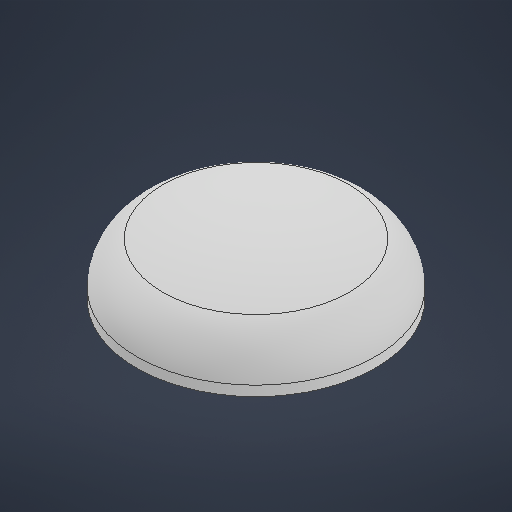
# Autodesk Inventor part: Fuel Cap Outlet
Saved by Autodesk Inventor 2026 (Build 300175050, 175E)
## iProperties
Created: 2026-03-18
Part Number: Fuel Cap Outlet
Material: Generic
Document SubType Name: Modeling
Designer: jackr
Density: 1 g/cm^3
Appearance: Default
Author: jackr
Autodesk Inventor part; units mm, degrees
ref_plane "YZ Plane" through (0, 0, 0) normal (1, 0, 0) x (0, 1, 0)
ref_plane "XZ Plane" through (0, 0, 0) normal (0, 1, 0) x (-1, 0, 0)
ref_plane "XY Plane" through (0, 0, 0) normal (0, 0, 1) x (1, 0, 0)
sketch "Sketch1" plane through (0, 0, 0) normal (0, 0, 1) x (1, 0, 0)
  arc A0 (0, 81.5967) -> (-112.679, 54.6437) centre (0, -167.4113) ccw
  arc A1 (-112.679, 54.6437) -> (-138.43, 12.7) centre (-91.3952, 12.7) ccw
  line L0 (-138.43, 12.7) -> (-138.43, 0)
  line L1 (-138.43, 0) -> (-152.4922, 0)
  line L2 (-152.4922, 0) -> (-152.4922, 12.7)
  line L3 (0, 95.6589) -> (0, 81.5967)
  line L4 (0, -183.3293) -> (0, 194.7967) projected
  line L5 (-182.128, 12.7) -> (-119.505, 12.7) construction
  line L6 (-218.5536, 0) -> (36.4256, 0) projected
  arc A2 (-119.0423, 67.1838) -> (-152.4922, 12.7) centre (-91.3952, 12.7) ccw
  arc A3 (0, 95.6589) -> (-119.0423, 67.1838) centre (0, -167.4113) ccw
  point P0 (-145.4611, 0)
  dimension "Inner_D" = 138.43
  dimension "Thickness" = 14.0622
  dimension "Skirt_Length" = 12.7
  dimension "Knuckle" = 47.0348
  dimension "Crown" = 249.008
  dimension "Thickness_Top" = 14.0622
  dimension "Outside_Knuckle" = 61.0971
  constraints: 10 end point, 8 point on circle, 4 centre point, 4 tangent, 2 collinear, 2 line through centre, 2 perpendicular, 2 point on line, 2 vertical, 1 horizontal, 1 midpoint
  measures "Inner_D" distance between parallel lines of L4 L0
  measures "Thickness" distance of L0.end L1.end
  measures "Skirt_Length" distance from line of point (-145.461, 0) L5
  measures "Knuckle" radius of A1
  measures "Crown" radius of A0
  measures "Thickness_Top" distance of L3.start L3.end
  measures "Outside_Knuckle" radius of A2
revolve "Revolution2" add sketch "Sketch1" angle 360 about axis through (0, -10, 0) along (0, 1, 0) contours A0 A1 L0 L1 L2 A2 A3 L3
equation "\"Outlet_Cap_Wall_Thickness\" = 14.06223"
body "Solid2"
